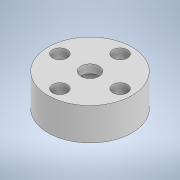
# Autodesk Inventor part: GoBilda Mech Hub 0500 Hex
Saved by Autodesk Inventor 2022 (Build 260153000, 153)
## iProperties
Created: 2021-12-21
Part Number: GoBilda Mech Hub 0500 Hex
Material: Generic
Document SubType Name: Modeling
Designer: TakeHomePC
Density: 1 g/cm^3
Appearance: Default
Author: TakeHomePC
Autodesk Inventor part; units mm, degrees
ref_plane "YZ Plane" through (0, 0, 0) normal (1, 0, 0) x (0, 1, 0)
ref_plane "XZ Plane" through (0, 0, 0) normal (0, 1, 0) x (-1, 0, 0)
ref_plane "XY Plane" through (0, 0, 0) normal (0, 0, 1) x (1, 0, 0)
sketch "Sketch1" plane through (0, 0, 0) normal (0, 1, 0) x (-1, 0, 0)
  circle A0 centre (11.3137, 0) radius 2.75
  circle A1 centre (0, 0) radius 15.739
  line L0 (0, -7.5575) -> (-6.545, -3.7788)
  line L1 (-6.545, -3.7788) -> (-6.545, 3.7788)
  line L2 (-6.545, 3.7788) -> (0, 7.5575)
  line L3 (0, 7.5575) -> (6.545, 3.7788)
  line L4 (6.545, 3.7788) -> (6.545, -3.7788)
  line L5 (6.545, -3.7788) -> (0, -7.5575)
  circle A2 centre (0, 11.3137) radius 2.75
  circle A3 centre (-11.3137, 0) radius 2.75
  circle A4 centre (0, -11.3137) radius 2.75
  circle A5 centre (0, 0) radius 3.4
  point P0 (0, 0)
  dimension "d0" = 31.478
  dimension "d3" = 13.09
  dimension "d4" = 5.5
  dimension "d7" = 360
  dimension "d11" = 6.8
  constraints: 12 end point, 6 centre point, 3 coincident, 22 other
  measures "d0" diameter of A1
  measures "d3" distance between parallel lines of L4 L1
  measures "d4" diameter of A0
  measures "d11" diameter of A5
extrude "Extrusion1" add sketch "Sketch1" along normal blind 9 contours A1
extrude "Extrusion2" add sketch "Sketch1" along normal blind 3.175 from surface at 9 contours A1 | L0 L1 L2 L3 L4 L5
body "Solid1"
